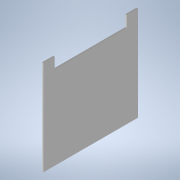
# Autodesk Inventor part: Frame
Saved by Autodesk Inventor 2022 (Build 260153000, 153)
## iProperties
Created: 2022-02-12
Part Number: Frame
Material: Generic
Document SubType Name: Modeling
Designer: ultra
Density: 1 g/cm^3
Appearance: Default
Author: ultra
Autodesk Inventor part; units mm, degrees
ref_plane "YZ Plane" through (0, 0, 0) normal (1, 0, 0) x (0, 1, 0)
ref_plane "XZ Plane" through (0, 0, 0) normal (0, 1, 0) x (-1, 0, 0)
ref_plane "XY Plane" through (0, 0, 0) normal (0, 0, 1) x (1, 0, 0)
sketch "Sketch1" plane through (0, 0, 0) normal (1, 0, 0) x (0, 1, 0)
  line L0 (0, 0) -> (321.6656, 0)
  line L1 (321.6656, 0) -> (321.6656, 321.6656)
  line L2 (321.6656, 321.6656) -> (0, 321.6656)
  line L3 (0, 321.6656) -> (0, 0)
  dimension "d0" = 321.6656
  dimension "d1" = 321.6656
  constraints: 8 end point, 2 parallel, 1 horizontal, 1 perpendicular
  measures "d0" distance of L2.end L1.end
  measures "d1" distance of L1.end L0.end
extrude "Extrusion1" add sketch "Sketch1" along normal blind 4.7752
sketch "Sketch3" plane through (0, 0, 0) normal (-1, 0, 0) x (0, 0, 1)
  line L0 (0, 321.6656) -> (321.6656, 321.6656) projected
  line L1 (321.6656, 321.6656) -> (321.6656, 0) projected
  line L2 (0, 321.6656) -> (321.6656, 321.6656) projected
  line L3 (321.6656, 321.6656) -> (283.5656, 321.6656)
  line L4 (283.5656, 321.6656) -> (283.5656, 283.5656)
  line L5 (283.5656, 283.5656) -> (321.6656, 283.5656)
  line L6 (321.6656, 283.5656) -> (321.6656, 321.6656)
  line L7 (321.6656, 321.6656) -> (321.6656, 0) projected
  line L8 (321.6656, 0) -> (283.5656, 0)
  line L9 (283.5656, 0) -> (283.5656, 38.1)
  line L10 (283.5656, 38.1) -> (321.6656, 38.1)
  line L11 (321.6656, 38.1) -> (321.6656, 0)
  line L12 (321.6656, 0) -> (0, 0) projected
  line L13 (0, 0) -> (38.1, 0)
  line L14 (38.1, 0) -> (38.1, 38.1)
  line L15 (38.1, 38.1) -> (0, 38.1)
  line L16 (0, 38.1) -> (0, 0)
  line L17 (0, 321.6656) -> (38.1, 321.6656)
  line L18 (38.1, 321.6656) -> (38.1, 283.5656)
  line L19 (38.1, 283.5656) -> (0, 283.5656)
  line L20 (0, 283.5656) -> (0, 321.6656)
  line L21 (283.5656, 321.6656) -> (38.1, 321.6656)
  line L22 (38.1, 321.6656) -> (38.1, 283.5656)
  line L23 (38.1, 283.5656) -> (283.5656, 283.5656)
  line L24 (283.5656, 283.5656) -> (283.5656, 321.6656)
  line L25 (321.6656, 283.5656) -> (283.5656, 283.5656)
  line L26 (283.5656, 283.5656) -> (283.5656, 38.1)
  line L27 (283.5656, 38.1) -> (321.6656, 38.1)
  line L28 (321.6656, 38.1) -> (321.6656, 283.5656)
  line L29 (38.1, 38.1) -> (0, 38.1)
  line L30 (0, 38.1) -> (0, 283.5656)
  line L31 (0, 283.5656) -> (38.1, 283.5656)
  line L32 (38.1, 283.5656) -> (38.1, 38.1)
  line L33 (38.1, 38.1) -> (283.5656, 38.1)
  line L34 (283.5656, 38.1) -> (283.5656, 0)
  line L35 (283.5656, 0) -> (38.1, 0)
  line L36 (38.1, 0) -> (38.1, 38.1)
  line L37 (321.6656, 283.5656) -> (283.5656, 245.4656)
  line L38 (321.6656, 283.5656) -> (375.5471, 283.5656) construction
  line L39 (283.5656, 245.4656) -> (283.5656, 321.6656)
  line L40 (283.5656, 321.6656) -> (245.4656, 283.5656)
  line L41 (283.5656, 321.6656) -> (337.4471, 321.6656) construction
  line L42 (38.1, 321.6656) -> (76.2, 283.5656)
  line L43 (38.1, 321.6656) -> (91.9815, 321.6656) construction
  line L44 (0, 283.5656) -> (38.1, 245.4656)
  line L45 (0, 283.5656) -> (53.8815, 283.5656) construction
  line L46 (0, 38.1) -> (38.1, 76.2)
  line L47 (0, 38.1) -> (53.8815, 38.1) construction
  line L48 (38.1, 0) -> (76.2, 38.1)
  line L49 (38.1, 0) -> (91.9815, 0) construction
  line L50 (321.6656, 38.1) -> (283.5656, 76.2)
  line L51 (321.6656, 38.1) -> (375.5471, 38.1) construction
  line L52 (283.5656, 0) -> (245.4656, 38.1)
  line L53 (283.5656, 0) -> (337.4471, 0) construction
  dimension "d14" = 38.1
  dimension "d15" = 38.1
  dimension "d16" = 38.1
  dimension "d17" = 38.1
  dimension "d18" = 38.1
  dimension "d19" = 38.1
  dimension "d20" = 38.1
  dimension "d21" = 135
  dimension "d22" = 135
  dimension "d25" = 45
  dimension "d26" = 45
  dimension "d27" = 45
  dimension "d28" = 45
  dimension "d29" = 135
  dimension "d30" = 135
  constraints: 98 end point, 16 horizontal, 16 parallel, 9 point on line, 8 equal length, 8 perpendicular, 1 collinear
  measures "d14" distance of L5.end L4.end
  measures "d15" distance of L4.end L3.end
  measures "d16" distance of L8.end L9.end
  measures "d17" distance of L15.end L14.end
  measures "d18" distance of L14.end L13.end
  measures "d19" distance of L18.end L19.end
  measures "d20" distance of L17.end L18.end
  measures "d21" angle of L37 L38
  measures "d22" angle of L40 L41
  measures "d25" angle of L42 L43
  measures "d26" angle of L44 L45
  measures "d27" angle of L47 L46
  measures "d28" angle of L49 L48
  measures "d29" angle of L51 L50
  measures "d30" angle of L53 L52
extrude "Extrusion4" cut sketch "Sketch3" against normal blind 4.7752 contours L0 L40 L23 L42 | L44 L32 L46 L30 | L1 L50 L26 L37 | L48 L33 L52 L12
sketch "Sketch4" plane through (0, 0, 0) normal (-1, 0, 0) x (0, 0, 1)
  line L0 (321.6656, 0) -> (283.5656, 0) projected
  line L1 (321.6656, 38.1) -> (321.6656, 0) projected
  line L2 (321.6656, 321.6656) -> (321.6656, 283.5656) projected
  line L3 (283.5656, 321.6656) -> (321.6656, 321.6656) projected
  line L4 (0, 321.6656) -> (38.1, 321.6656) projected
  line L5 (0, 283.5656) -> (0, 321.6656) projected
  line L6 (0, 0) -> (0, 38.1) projected
  line L7 (38.1, 0) -> (0, 0) projected
  line L8 (245.4656, 283.5656) -> (283.5656, 321.6656) projected
  line L9 (283.5656, 321.6656) -> (321.6656, 283.5656)
  line L10 (0, 283.5656) -> (0, 321.6656) projected
  line L11 (38.1, 321.6656) -> (0, 283.5656)
  line L12 (0, 38.1) -> (38.1, 0)
  line L13 (283.5656, 0) -> (321.6656, 38.1)
  constraints: 8 end point, 2 perpendicular, 1 point on line
extrude "Extrusion5" cut sketch "Sketch4" against normal blind 4.7752
fillet "Fillet1" radius 6.35 16 edges at (2.3876, 283.5656, 0) (2.3876, 321.6656, 38.1) (2.3876, 38.1, 0) (2.3876, 76.2, 38.1) (2.3876, 0, 38.1) (2.3876, 283.5656, 76.2) (2.3876, 283.5656, 245.4656) (2.3876, 321.6656, 283.5656) (2.3876, 283.5656, 321.6656) (2.3876, 76.2, 283.5656) (2.3876, 245.4656, 283.5656) (2.3876, 0, 283.5656) (2.3876, 38.1, 321.6656) (2.3876, 38.1, 76.2) (2.3876, 38.1, 245.4656) (2.3876, 245.4656, 38.1)
body "Solid1"
